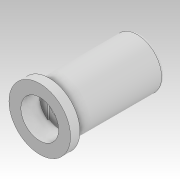
# Autodesk Inventor part: HD_BearingShaft2
Saved by Autodesk Inventor 2020 (Build 240168000, 168)
## iProperties
Created: 2021-03-21
Part Number: HD_BearingShaft2
Material: Generic
Document SubType Name: Modeling
Designer: DDeGo
Density: 1 g/cm^3
Appearance: Default
Author: DDeGo
Autodesk Inventor part; units mm, degrees
ref_plane "YZ Plane" through (0, 0, 0) normal (1, 0, 0) x (0, 1, 0)
ref_plane "XZ Plane" through (0, 0, 0) normal (0, 1, 0) x (-1, 0, 0)
ref_plane "XY Plane" through (0, 0, 0) normal (0, 0, 1) x (1, 0, 0)
sketch "Sketch1" plane through (0, 0, 0) normal (1, 0, 0) x (0, 1, 0)
  line L0 (0, 0) -> (1.65, 0) construction
  line L1 (1.65, 0) -> (3, 0) construction
  line L2 (4.9, 0) -> (4.9, -1.5)
  line L3 (4.9, -1.5) -> (3.9, -1.5)
  line L4 (3.9, -1.5) -> (3.9, -16)
  line L5 (3.9, -16) -> (1.7, -16)
  line L6 (1.7, -16) -> (1.7, -3)
  line L7 (0, 0) -> (0, -13.7466) construction
  line L8 (3, 0) -> (3, -3)
  line L9 (3, -3) -> (1.7, -3)
  line L10 (3, 0) -> (4.9, 0)
  dimension "d0" = 1.7
  dimension "d1" = 3.9
  dimension "d2" = 1
  dimension "d3" = 1.5
  dimension "d4" = 14.5
  dimension "d6" = 3
  dimension "d7" = 3
  constraints: 22 end point, 7 perpendicular, 3 vertical, 1 horizontal, 1 point on line
  measures "d0" distance between parallel lines of L7 L6
  measures "d1" distance between parallel lines of L7 L4
  measures "d2" distance between parallel lines of L4 L2
  measures "d3" distance between parallel lines of L1 L3
  measures "d4" distance of L3.end L4.end
  measures "d6" distance between parallel lines of L7 L8
  measures "d7" distance between parallel lines of L1 L9
revolve "Revolution1" add sketch "Sketch1" angle 360 about axis through (0, 0, 0) along (0, 0, -1)
fillet "Fillet1" radius 0.5 2 edges at (0, -1.7, -16) (0, -3.9, -16)
sketch "Sketch2" plane through (0, 0, -3) normal (0, 0, 1) x (1, 0, 0)
  circle A0 centre (0, 0) radius 3 projected
  line L0 (-1.7, 2.4718) -> (1.7, 2.4718) construction
  line L1 (1.7, 2.4718) -> (1.7, -2.4718)
  line L2 (1.7, -2.4718) -> (-1.7, -2.4718) construction
  line L3 (-1.7, -2.4718) -> (-1.7, 2.4718)
  circle A1 centre (0, 0) radius 1.7 projected
  point P0 (-1.7, 0)
  point P1 (1.7, 0)
  constraints: 8 end point, 3 point on circle, 2 parallel, 1 horizontal, 1 perpendicular, 1 tangent
extrude "Extrusion1" cut sketch "Sketch2" against normal blind 0.2 contours L1 A1 L3 A0 | A0 L3 A1 L1
body "Solid1"
